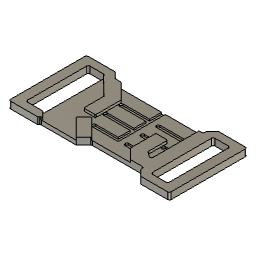
はるまさ_バックル_mk1 v6 (Autodesk Fusion 360 design; units mm, degrees)
Autodesk Fusion 360 part; units mm, degrees
sketch "スケッチ1" plane through (0, 0, 0) normal (0, 0, 1) x (1, 0, 0)
  line L0 (-47.5, 23) -> (47.5, 23)
  line L1 (47.5, 23) -> (47.5, -23)
  line L2 (47.5, -23) -> (-47.5, -23)
  line L3 (-47.5, -23) -> (-47.5, 23)
  line L4 (0, -23) -> (0, 23) construction
  line L5 (-47.5, 0) -> (47.5, 0) construction
  line L6 (-42, 18.5) -> (-32, 18.5)
  line L7 (-32, 18.5) -> (-32, -18.5)
  line L8 (-32, -18.5) -> (-42, -18.5)
  line L9 (-42, -18.5) -> (-42, 18.5)
  line L10 (42, 18.5) -> (32, 18.5)
  line L11 (42, -18.5) -> (42, 18.5)
  line L12 (32, 18.5) -> (32, -18.5)
  line L13 (32, -18.5) -> (42, -18.5)
  line L14 (-30.5, 23) -> (-27, 19.5)
  line L15 (-27, 19.5) -> (-27, 17.5)
  line L16 (-27, 17.5) -> (4, 17.5)
  line L17 (-30.5, -23) -> (-27, -19.5)
  line L18 (-27, -19.5) -> (-27, -17.5)
  line L19 (-27, -17.5) -> (-24.5, -17.5)
  line L20 (-24.5, -17.5) -> (-24.5, 11.5)
  line L21 (-19, 17.5) -> (-13, 11.5)
  line L22 (-13, 11.5) -> (-13, -3.5)
  line L23 (-13, -3.5) -> (-20, -3.5)
  line L24 (-24.5, -17.5) -> (21.5, -17.5)
  line L25 (30.5, -23) -> (27, -19.5)
  line L26 (27, -19.5) -> (23.5, -19.5)
  line L27 (-3.5, -17.5) -> (-3.5, 17.5) construction
  line L28 (-4.6, -17.5) -> (-4.6, 10.4)
  line L29 (-24.5, -10.4) -> (-7.6, -10.4)
  line L30 (-7.6, -10.4) -> (-7.6, -8.2)
  line L31 (-7.6, -8.2) -> (-24.5, -8.2)
  line L32 (-7.6, -1.1) -> (-7.6, 1.1)
  line L33 (-7.6, 8.2) -> (-7.6, 10.4)
  line L34 (-20, -3.5) -> (-20, 8.2)
  line L35 (-20, 8.2) -> (-24.5, 11.5)
  line L36 (-7.6, 10.4) -> (-13, 10.4)
  line L37 (-23, 10.4) -> (-24.5, 10.4)
  line L38 (-24.5, 8.2) -> (-20, 8.2)
  line L39 (-13, 8.2) -> (-7.6, 8.2)
  line L40 (21.5, -17.5) -> (23.5, -19.5)
  line L41 (-2.4, -10.4) -> (14.4, -10.4)
  line L42 (-2.4, -8.2) -> (14.4, -8.2)
  line L43 (-2.4, -1.1) -> (14.4, -1.1)
  line L44 (-2.4, 1.1) -> (14.4, 1.1)
  line L45 (-2.4, 1.1) -> (-2.4, 8.2)
  line L46 (-2.4, -17.5) -> (-2.4, -10.4)
  line L47 (-2.4, -8.2) -> (-2.4, -1.1)
  line L48 (21.5, -17.5) -> (14.4, -10.4)
  line L49 (14.4, -10.4) -> (14.4, 4.85)
  line L50 (14.4, 4.85) -> (21.4, 4.85)
  line L51 (21.4, 4.85) -> (21.4, -7.15)
  line L52 (4, 17.5) -> (14.45, 7.05)
  line L53 (-4.6, 10.4) -> (11.1, 10.4)
  line L54 (-2.4, 8.2) -> (13.3, 8.2)
  line L55 (4, 17.5) -> (8.5962, 22.0962)
  line L56 (8.5962, 22.0962) -> (19.0462, 11.6462)
  line L57 (14.45, 7.05) -> (19.0462, 11.6462)
  line L58 (30.5, 23) -> (29.5962, 22.0962)
  line L59 (8.5962, 22.0962) -> (29.5962, 22.0962)
  line L60 (32, 18.5) -> (28.4038, 22.0962)
  line L61 (-7.6, 1.1) -> (-13, 1.1)
  line L62 (-20, 1.1) -> (-24.5, 1.1)
  line L63 (-24.5, -1.1) -> (-20, -1.1)
  line L64 (-13, -1.1) -> (-7.6, -1.1)
  line L65 (21.4, -7.15) -> (32, -17.5)
  dimension "d2" = 95
  dimension "d3" = 46
  dimension "d4" = 4.5
  dimension "d5" = 4.5
  dimension "d6" = 5.5
  dimension "d7" = 10
  dimension "d8" = 17
  dimension "d9" = 3.5
  dimension "d10" = 45
  dimension "d11" = 2
  dimension "d12" = 31
  dimension "d13" = 7.5
  dimension "d14" = 6
  dimension "d15" = 8
  dimension "d16" = 45
  dimension "d17" = 6
  dimension "d18" = 15
  dimension "d19" = 7
  dimension "d21" = 46
  dimension "d23" = 3.5
  dimension "d24" = 21
  dimension "d25" = 7.1
  dimension "d26" = 1.1
  dimension "d27" = 9.3
  dimension "d28" = 3
  dimension "d29" = 7.1
  dimension "d30" = 2.2
  dimension "d31" = 3
  dimension "d32" = 2.2
  dimension "d33" = 7.1
  dimension "d34" = 2.2
  dimension "d35" = 3
  dimension "d36" = 7.1
  dimension "d37" = 7.1
  dimension "d38" = 2.2
  dimension "d39" = 7.1
  dimension "d40" = 2.2
  dimension "d41" = 15.25
  dimension "d42" = 7
  dimension "d43" = 12
  dimension "d46" = 135
  dimension "d47" = 2.2
  dimension "d49" = 6.5
  dimension "d50" = 45
  dimension "d52" = 135
  dimension "d92" = 1
  constraint horizontal L0
  constraint vertical L1
  constraint horizontal L2
  constraint vertical L3
  constraint midpoint L2 L4.start
  constraint midpoint L0 L4.end
  constraint midpoint L3 L5.start
  constraint midpoint L1 L5.end
  constraint midpoint origin L4
  constraint horizontal L6
  constraint vertical L7
  constraint horizontal L8
  constraint vertical L9
  constraint symmetric L4 L6.start L10.start
  constraint symmetric L4 L6.end L10.end
  constraint symmetric L4 L7.end L12.end
  constraint symmetric L4 L8.end L11.start
  constraint coincident L0 L14.start
  constraint vertical L15
  constraint perpendicular L15 L16
  constraint symmetric L5 L14.start L17.start
  constraint symmetric L5 L14.end L17.end
  constraint symmetric L5 L15.end L18.end
  constraint perpendicular L18 L19
  constraint perpendicular L5 L20
  constraint coincident L16 L21.start
  constraint perpendicular L6 L22
  constraint perpendicular L22 L23
  constraint perpendicular L20 L24
  constraint symmetric L4 L17.start L25.start
  constraint symmetric L4 L17.end L25.end
  constraint parallel L2 L26
  constraint perpendicular L24 L27
  constraint coincident L24 L27.start
  constraint coincident L16 L27.end
  constraint coincident L24 L28.start
  constraint perpendicular L5 L28
  constraint perpendicular L5 L46
  constraint coincident L20 L29.start
  constraint perpendicular L20 L29
  constraint perpendicular L29 L30
  constraint coincident L20 L31.end
  constraint perpendicular L20 L31
  constraint coincident L20 L63.start
  constraint perpendicular L22 L63
  constraint perpendicular L5 L32
  constraint coincident L20 L62.end
  constraint perpendicular L20 L61
  constraint coincident L20 L38.start
  constraint perpendicular L22 L38
  constraint perpendicular L33 L38
  constraint coincident L20 L37.end
  constraint perpendicular L20 L36
  constraint perpendicular L34 L38
  constraint coincident L22 L36.end
  constraint coincident L35 L37.start
  constraint collinear L36 L37
  constraint coincident L22 L39.start
  constraint collinear L38 L39
  constraint perpendicular L12 L53
  constraint perpendicular L12 L54
  constraint perpendicular L12 L41
  constraint coincident L42.start L46
  constraint perpendicular L12 L42
  constraint perpendicular L12 L43
  constraint coincident L44.start L46
  constraint perpendicular L12 L44
  constraint collinear L45 L46
  constraint collinear L46 L47
  constraint parallel L40 L48
  constraint perpendicular L44 L49
  constraint coincident L49 L44.end
  constraint coincident L49 L43.end
  constraint coincident L49 L42.end
  constraint perpendicular L49 L50
  constraint perpendicular L50 L51
  constraint coincident L52 L53.end
  constraint coincident L52 L54.end
  constraint perpendicular L52 L55
  constraint perpendicular L55 L56
  constraint equal L52 L56
  constraint symmetric L4 L14.start L58.start
  constraint horizontal L59
  constraint coincident L59 L60.end
  constraint coincident L22 L61.end
  constraint coincident L34 L62.start
  constraint collinear L61 L62
  constraint coincident L34 L63.end
  constraint coincident L22 L64.start
  constraint collinear L63 L64
  constraint coincident L12 L65.end
  measures "d2" distance of L0.start L0.end
  measures "d3" distance of L0.start L2.end
  measures "d4" distance of L0 L6
  measures "d5" distance of L2 L8
  measures "d6" distance of L3 L9
  measures "d7" distance of L6.start L6.end
  measures "d8" distance of L0.start L14.start
  measures "d9" distance of L0 L14.end
  measures "d10" angle of L0 L14
  measures "d11" distance of L14.end L15.end
  measures "d12" distance of L15.end L16.end
  measures "d13" distance of L7 L19.end
  measures "d14" distance of L16 L20.end
  measures "d15" distance of L15.end L21.start
  measures "d16" angle of L16 L21
  measures "d17" distance of L16 L21.end
  measures "d18" distance of L21.end L22.end
  measures "d19" distance of L22.end L23.end
  measures "d21" distance of L19.end L24.end
  measures "d23" distance of L25.end L26.end
  measures "d24" distance of L20 L27
  measures "d25" distance of L16 L28.end
  measures "d26" distance of L27 L28
  measures "d27" distance of L16 L45.end
  measures "d28" distance of L28 L29.end
  measures "d29" distance of L24 L29
  measures "d30" distance of L29.end L30.end
  measures "d31" distance of L28 L32.start
  measures "d32" distance of L32.start L32.end
  measures "d33" distance of L31 L63
  measures "d34" distance of L33.start L33.end
  measures "d35" distance of L28 L33
  measures "d36" distance of L38 L61
  measures "d37" distance of L24 L41
  measures "d38" distance of L41 L42
  measures "d39" distance of L42 L43
  measures "d40" distance of L43 L44
  measures "d41" distance of L41.end L49.end
  measures "d42" distance of L49.end L50.end
  measures "d43" distance of L50.end L51.end
  measures "d46" angle of L16 L52
  measures "d47" distance of L50 L52.end
  measures "d49" distance of L16.end L55.end
  measures "d50" angle of L0 L58
  measures "d52" angle of L10 L60
  measures "d92" distance of L13 L65.end
extrude "押し出し2" add sketch "スケッチ1" along normal blind 4 contours L0 L2 L3 L14 L15 L16 L17 L18 L19 L20 L21 L22 L23 L34 L35 | L0 L1 L2 L10 L11 L12 L13 L25 L26 L40 L48 L49 L50 L51 L58 L59 L60 L65 | L52 L55 L56 L57 makes body 1 at (-29.5, 3.8333, 0) makes body 2 at (9.0154, 15.5487, 0) makes body 3 at (16.7333, -4.2333, 0)
extrude "押し出し6" add sketch "スケッチ1" along normal blind 2.5 contours L12 L44 L45 L49 L50 L51 L52 L54 L56 L57 L59 L60 L65 | L16 L20 L21 L22 L23 L24 L28 L29 L30 L31 L32 L33 L34 L36 L39 L52 L53 L61 L63 L64 | L24 L41 L46 L48 | L42 L43 L47 L49 | L20 L34 L38 L62 | L20 L35 L37 L38 | L20 L35 L37 bodies 1 2 3
extrude "押し出し7" add sketch "スケッチ1" along normal blind 1.5 contours L24 L28 L41 L42 L43 L44 L45 L46 L47 L49 L52 L53 L54 | L22 L33 L36 L39 | L20 L29 L30 L31 | L22 L32 L61 L64 | L20 L34 L62 L63 bodies 1
fillet "フィレット1" radius 1 1 edges at (-24.5, 11.5, 3.25) on bodies 1
fillet "フィレット2" radius 1 1 edges at (-20, 8.2, 3.25) on bodies 1
fillet "フィレット3" radius 1 1 edges at (13.3, 8.2, 2) on bodies 1
fillet "フィレット4" radius 1 1 edges at (11.1, 10.4, 2) on bodies 1
fillet "フィレット5" radius 1 1 edges at (14.4, 1.1, 2) on bodies 1
fillet "フィレット6" radius 1 2 edges at (14.4, -1.1, 2) (14.4, -8.2, 2) on bodies 1
ref_plane "作業平面1" through (9.55, -13.95, 2.5) normal (0, 0, 1) x (1, 0, 0)
split_face "面を分割1" 1 faces at (14.4, -1.8833, 3.5) by plane through (9.55, -13.95, 2.5) normal (0, 0, 1) on bodies 1
fillet "フィレット7" radius 1 1 edges at (14.4, -10.4, 2) on bodies 1
fillet "フィレット8" radius 1 1 edges at (-4.6, 10.4, 2) on bodies 1
fillet "フィレット9" radius 1 12 edges at (-13, -1.1, 2) (-13, 1.1, 2) (-13, 10.4, 2) (-13, 8.2, 2) (-7.6, 8.2, 2) (-7.6, 10.4, 2) (-7.6, 1.1, 2) (-7.6, -1.1, 2) (-7.6, -10.4, 2) (-7.6, -8.2, 2) (-24.5, -10.4, 2) (-24.5, -8.2, 2) on bodies 1
fillet "フィレット10" radius 1 4 edges at (-20, 1.1, 2) (-20, -1.1, 2) (-24.5, -1.1, 2) (-24.5, 1.1, 2) on bodies 1
fillet "フィレット11" radius 1 3 edges at (-27, -17.5, 2) (21.5, -17.5, 1.25) (27, -19.5, 2) on bodies 1
fillet "フィレット12" radius 1 3 edges at (29.5962, 22.0962, 2) (4, 17.5, 1.25) (-27, 17.5, 2) on bodies 1
split_face "面を分割2" 1 faces at (38.6667, 18.5, 2.1667) by plane through (9.55, -13.95, 2.5) normal (0, 0, 1) on bodies 1
fillet "フィレット13" radius 1 5 edges at (32, 18.5, 1.25) (42, 18.5, 1.25) (42, 18.5, 3.25) (42, -18.5, 2) (32, -18.5, 2) on bodies 1
fillet "フィレット14" radius 1 4 edges at (-32, 18.5, 2) (-42, 18.5, 2) (-42, -18.5, 2) (-32, -18.5, 2) on bodies 1
fillet "フィレット15" radius 1 4 edges at (47.5, -23, 2) (47.5, 23, 2) (-47.5, 23, 2) (-47.5, -23, 2) on bodies 1
fillet "フィレット16" radius 0.5 1 edges at (28.4038, 22.0962, 3.25) on bodies 1
fillet "フィレット17" radius 0.5 4 edges at (21.4, 4.85, 3.25) (14.4, 4.85, 3.25) (19.0462, 11.6462, 3.25) (14.45, 7.05, 3.25) on bodies 1
fillet "フィレット18" radius 0.5 2 edges at (-13, -3.5, 3.25) (-20, -3.5, 3.25) on bodies 1
move_body "移動1" bodies 1 to x (-1, 0, 0) y (0, -1, 0) z (0, 0, 1) at (-95, -46, 0)
move_body "移動2" bodies 1 to x (1, 0, 0) y (0, 1, 0) z (0, 0, 1) at (107, 0, 0)
equation "d5 = d4"
equation "d9 = d4 - 1 mm"
equation "d17 = d14"
equation "d27 = d25 + 2.2 mm"
equation "d31 = d28"
equation "d32 = d30"
equation "d33 = d29"
equation "d34 = d30"
equation "d35 = d28"
equation "d36 = d33"
equation "d37 = d29"
equation "d38 = d30"
equation "d39 = d29"
